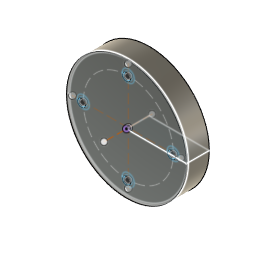
Fan cover (Autodesk Fusion 360 design; units mm, degrees)
Autodesk Fusion 360 part; units mm, degrees
sketch "Sketch1" plane through (0, 0, 0) normal (0, 0, 1) x (1, 0, 0)
  line L0 (0, 17) -> (0, -15) construction
  line L1 (0, 0) -> (40, 0)
  line L2 (0, 0) -> (0, 15)
  line L3 (0, 15) -> (40, 15)
  line L4 (40, 0) -> (40, 15)
  dimension "d1" = 40
  dimension "d2" = 15
  dimension "d3" = 40
  constraint vertical L0
  constraint coincident L1.start L2.start
  constraint perpendicular L0 L1
  constraint perpendicular L1 L2
  constraint perpendicular L0 L3
  measures "d1" distance of L1.start L1.end
  measures "d2" distance of L1.start L2.end
  measures "d3" distance of L2.end L3.end
revolve "Revolve1" add sketch "Sketch1" angle 360 about axis through (0, 17, 0) along (0, -1, 0)
shell "Shell1" thickness 1.2 removed faces 1 at (7.7208, 15, -6.4944)
sketch "Sketch2" plane through (0, 1.2, 0) normal (0, 1, 0) x (-1, 0, 0)
  circle A0 centre (0, 0) radius 38.8
  circle A1 centre (0, 0) radius 30 construction
  line L0 (0, 37) -> (0, -35) construction
  line L1 (-35, 0) -> (37.2005, 0) construction
  circle A2 centre (0, 30) radius 2.6
  circle A3 centre (-30, 0) radius 2.6
  circle A4 centre (30, 0) radius 2.6
  circle A5 centre (0, -30) radius 2.6
  circle A6 centre (-30, 0) radius 4
  circle A7 centre (0, -30) radius 4
  circle A8 centre (30, 0) radius 4
  circle A9 centre (0, 30) radius 4
  dimension "d6" = 60
  dimension "d7" = 72
  dimension "d8" = 72.2005
  dimension "d9" = 5.2
  dimension "d10" = 5.2
  dimension "d11" = 5.2
  dimension "d12" = 5.2
  dimension "d13" = 8
  dimension "d14" = 8
  dimension "d15" = 8
  dimension "d16" = 8
  constraint coincident A0.centre A1.centre
  constraint vertical L0
  constraint horizontal L1
  constraint coincident L0 A2.centre
  constraint coincident A1 A2.centre
  constraint coincident L1 A3.centre
  constraint coincident A1 A3.centre
  constraint coincident L1 A4.centre
  constraint coincident A1 A4.centre
  constraint coincident L0 A5.centre
  constraint coincident A1 A5.centre
  constraint concentric A3 A6
  constraint concentric A5 A7
  constraint concentric A4 A8
  constraint concentric A2 A9
  measures "d6" diameter of A1
  measures "d7" distance of L0.start L0.end
  measures "d8" distance of L1.start L1.end
  measures "d9" diameter of A2
  measures "d10" diameter of A3
  measures "d11" diameter of A4
  measures "d12" diameter of A5
  measures "d13" diameter of A6
  measures "d14" diameter of A7
  measures "d15" diameter of A8
  measures "d16" diameter of A9
extrude "Extrude13" add sketch "Sketch2" along normal blind 13 contours A6 | A7 | A8 | A9
extrude "Extrude11" cut sketch "Sketch2" against normal blind 5 contours A2 | A3 | A4 | A5
sketch "Sketch8" plane through (0, 1.2, 0) normal (0, 1, 0) x (-1, 0, 0)
  circle A0 centre (0, 0) radius 39
  circle A1 centre (0, 0) radius 40
  dimension "d39" = 78
  dimension "d40" = 80
  constraint coincident A0.centre A1.centre
  constraint concentric A0 A1
  measures "d39" diameter of A0
  measures "d40" diameter of A1
extrude "Extrude9" cut sketch "Sketch8" along normal blind 14
extrude "Extrude10" add sketch "Sketch8" along normal blind 14
